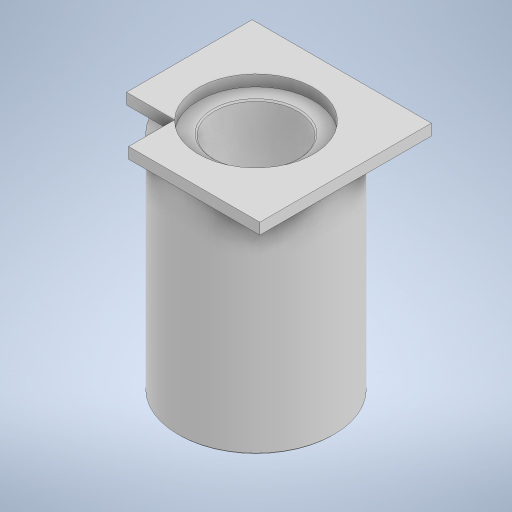
# Autodesk Inventor part: Wheel Washer
Saved by Autodesk Inventor 2024 (Build 280153000, 153)
## iProperties
Created: 2023-10-18
Part Number: Wheel Washer
Material: Generic
Document SubType Name: Modeling
Designer: luke.macenski3281
Density: 1 g/cm^3
Appearance: Default
Author: luke.macenski3281
Autodesk Inventor part; units mm, degrees
ref_plane "YZ Plane" through (0, 0, 0) normal (1, 0, 0) x (0, 1, 0)
ref_plane "XZ Plane" through (0, 0, 0) normal (0, 1, 0) x (-1, 0, 0)
ref_plane "XY Plane" through (0, 0, 0) normal (0, 0, 1) x (1, 0, 0)
sketch "Sketch1" plane through (0, 0, 0) normal (0, 1, 0) x (-1, 0, 0)
  point P0 (0, 0)
sketch "Sketch2" plane through (0, 0, 0) normal (0, 1, 0) x (-1, 0, 0)
  circle A0 centre (0, 0) radius 17.78
  circle A1 centre (0, 0) radius 9.525
  dimension "d0" = 35.56
  dimension "d1" = 19.05
  constraints: 2 centre point, 2 coincident
  measures "d0" diameter of A0
  measures "d1" diameter of A1
extrude "Extrusion1" add sketch "Sketch2" along normal blind 50.8
chamfer "Chamfer1" distance 0.3175 angle 45 2 edges at (9.525, 50.8, 0) (17.78, 0, 0)
sketch "Sketch3" plane through (0, 50.8, 0) normal (0, 1, 0) x (1, 0, 0)
  line L0 (-20.433, 19.5533) -> (20.433, 19.5533)
  line L1 (20.433, 19.5533) -> (20.433, -19.5533)
  line L2 (20.433, -19.5533) -> (-20.433, -19.5533)
  line L3 (-20.433, -19.5533) -> (-20.433, 19.5533)
  line L4 (-20.433, 19.5533) -> (20.433, -19.5533) construction
  line L5 (20.433, 19.5533) -> (-20.433, -19.5533) construction
  line L6 (-14.9596, 14.3155) -> (14.9596, 14.3155)
  line L7 (14.9596, 14.3155) -> (14.9596, -14.3155)
  line L8 (14.9596, -14.3155) -> (-14.9596, -14.3155)
  line L9 (-14.9596, -14.3155) -> (-14.9596, 14.3155)
  line L10 (-14.9596, 14.3155) -> (14.9596, -14.3155) construction
  line L11 (14.9596, 14.3155) -> (-14.9596, -14.3155) construction
  line L12 (-9.4862, -9.0778) -> (-20.433, -9.0778)
  line L13 (-20.433, -9.0778) -> (-20.433, -19.5533)
  line L14 (-20.433, -19.5533) -> (-9.4862, -19.5533)
  line L15 (-9.4862, -19.5533) -> (-9.4862, -9.0778)
  line L16 (-9.4862, -9.0778) -> (-20.433, -19.5533) construction
  line L17 (-20.433, -9.0778) -> (-9.4862, -19.5533) construction
  circle A0 centre (0, 0) radius 13.1299
  constraints: 36 end point, 6 midpoint, 6 parallel, 3 horizontal, 3 perpendicular, 1 coincident, 1 point on line, 3 other
extrude "Extrusion2" add sketch "Sketch3" along normal blind 2.54 contours L0 L1 L2 L15 L8 L7 L6 L9 L12 L3 | L9 L6 L7 L8 L15 L12
body "Solid1"
